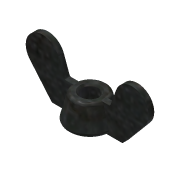
# Autodesk Inventor part: IntroToiLogic01_2015
Saved by Autodesk Inventor 2019.1 (Build 231200000, 200)
## iProperties
Created: 2015-07-09
Part Number: IntroToiLogic01_2015
Material: Steel
Document SubType Name: Modeling
Designer: MRT
Stock Number: Standard (in)
Density: 7.85 g/cm^3
Appearance: Plate
Mass: 5.82255 g
Surface Area: 9.55133 cm^2
Volume: 0.741726 cm^3
RuleStatus: InUse
TheMass: 0.013 lbmass
TheVolume: 741.726 millimeter^3
TheSurfArea: 955.133 millimeter^2
Author: MRT
Autodesk Inventor part; units mm, degrees
ref_plane "YZ Plane" through (0, 0, 0) normal (1, 0, 0) x (0, 1, 0)
ref_plane "XZ Plane" through (0, 0, 0) normal (0, 1, 0) x (-1, 0, 0)
ref_plane "XY Plane" through (0, 0, 0) normal (0, 0, 1) x (1, 0, 0)
sketch "Sketch1" plane through (0, 0, 0) normal (0, 0, 1) x (1, 0, 0)
  line L0 (0, 0) -> (0, 7)
  line L1 (0, 7) -> (-4.25, 7)
  line L2 (-4.25, 7) -> (-6, 0)
  line L3 (-6, 0) -> (0, 0)
  line L4 (0, 0) -> (0, -3.908269)
  dimension "BaseHt" = 7
  dimension "BaseTopDia" = 8.5
  dimension "BaseDia" = 12
  constraints: 10 end point, 1 parallel, 1 perpendicular, 1 point on line, 1 vertical
  measures "BaseHt" distance of L0.start L0.end
  measures "BaseTopDia" diameter of L1.end L4
  measures "BaseDia" diameter of L2.end L4
sketch "Sketch1 outline for Revolution1" plane through (0, 0, 0) normal (0, 0, 1) x (1, 0, 0)
  line L0 (-6, 0) -> (0, 0)
  line L1 (-4.25, 7) -> (-6, 0)
  line L2 (0, 7) -> (-4.25, 7)
  line L3 (0, 0) -> (0, 7)
revolve "Revolution1" add sketch "Sketch1 outline for Revolution1" angle 360 about axis through (0, 0, 0) along (0, -1, 0)
fillet "Fillet1" radius 0.85 2 edges at (4.25, 7, 0) (6, 0, 0)
sketch "Sketch2" plane through (0, 0, 0) normal (0, 0, 1) x (1, 0, 0)
  arc A0 (-5.735961, 1.056155) -> (-4.91134, 0) centre (-4.91134, 0.85) ccw
  line L0 (-5.735961, 1.056155) -> (-4.410961, 6.356155)
  arc A1 (-3.58634, 7) -> (-4.410961, 6.356155) centre (-3.58634, 6.15) ccw
  line L1 (-3.58634, 7) -> (3.58634, 7)
  arc A2 (4.410961, 6.356155) -> (3.58634, 7) centre (3.58634, 6.15) ccw
  line L2 (4.410961, 6.356155) -> (5.735961, 1.056155)
  arc A3 (4.91134, 0) -> (5.735961, 1.056155) centre (4.91134, 0.85) ccw
  line L3 (4.91134, 0) -> (-4.91134, 0)
  line L4 (-4.91134, 0) -> (-9.483336, 0)
  line L5 (-9.483336, 0) -> (-15.4472, 7.107456)
  arc A4 (-7.771383, 11.539091) -> (-15.4472, 7.107456) centre (-12, 10) ccw
  line L6 (-7.771383, 11.539091) -> (-6.119289, 7)
  line L7 (-6.119289, 7) -> (-3.58634, 7)
  line L8 (0, 0) -> (0, 7)
  dimension "d5" = 50
  dimension "d6" = 20
  dimension "WingNutRad" = 4.5
  dimension "WingNutHt" = 10
  dimension "WingNutCen" = 24
  constraints: 10 end point, 2 point on circle, 2 tangent, 1 centre point, 1 horizontal, 1 midpoint, 1 parallel
  measures "d5" angle of L4 L5
  measures "d6" angle of L8 L6
  measures "WingNutRad" radius of A4
  measures "WingNutHt" distance from line of L4 A4.centre
  measures "WingNutCen" diameter of A4.centre L8
sketch "Sketch2 outline for Extrusion1" plane through (0, 0, 0) normal (0, 0, 1) x (1, 0, 0)
  line L0 (-9.483336, 0) -> (-4.91134, 0)
  line L1 (-15.4472, 7.107456) -> (-9.483336, 0)
  arc A0 (-7.771383, 11.539091) -> (-15.4472, 7.107456) centre (-12, 10) ccw
  line L2 (-6.119289, 7) -> (-7.771383, 11.539091)
  line L3 (-3.58634, 7) -> (-6.119289, 7)
  arc A1 (-4.410961, 6.356155) -> (-3.58634, 7) centre (-3.58634, 6.15) cw
  line L4 (-5.735961, 1.056155) -> (-4.410961, 6.356155)
  arc A2 (-4.91134, 0) -> (-5.735961, 1.056155) centre (-4.91134, 0.85) cw
extrude "Extrusion1" add sketch "Sketch2 outline for Extrusion1" along normal mid plane 1.5
fillet "Fillet2" radius 0.425 2 edges at (-6.1193, 7, 0) (-9.4833, 0, 0)
mirror "Mirror1" about plane through (0, 0, 0) normal (1, 0, 0) of "Extrusion1", "Fillet2"
hole "Hole1" at (0, 7, 0) direction (0, -1, 0) diameter 4.5 end through all clearance for "Hex Head Cap Screw DIN EN 24017" size "M4" standard "DIN"
chamfer "Chamfer1" distance 0.45 angle 45 2 edges at (0, 7, -2.25) (0, 0, -2.25)
equation "\"d4\" = 0.1 * BaseTopDia"
equation "\"d12\" = 0.05 * BaseTopDia"
equation "\"d22\" = 0.1 * d15"
equation "\"d15\" = 4.5"
body "Solid1"
